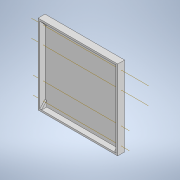
# Autodesk Inventor part: Bottom Base
Saved by Autodesk Inventor 2022 (Build 260153000, 153)
## iProperties
Created: 2022-04-03
Part Number: Bottom Base
Material: Generic
Document SubType Name: Modeling
Designer: Nick
Density: 1 g/cm^3
Appearance: Default
Author: Nick
Autodesk Inventor part; units mm, degrees
ref_plane "YZ Plane" through (0, 0, 0) normal (1, 0, 0) x (0, 1, 0)
ref_plane "XZ Plane" through (0, 0, 0) normal (0, 1, 0) x (-1, 0, 0)
ref_plane "XY Plane" through (0, 0, 0) normal (0, 0, 1) x (1, 0, 0)
sketch "Sketch1" plane through (0, 0, 0) normal (0, 0, 1) x (1, 0, 0)
  line L0 (0, 0) -> (292.1, 0)
  line L1 (292.1, 0) -> (292.1, 292.1)
  line L2 (292.1, 292.1) -> (0, 292.1)
  line L3 (0, 292.1) -> (0, 0)
  dimension "d11" = 292.1
  dimension "d12" = 292.1
  constraints: 8 end point, 2 parallel, 1 horizontal, 1 perpendicular
  measures "d11" distance of L2.end L1.end
  measures "d12" distance of L1.end L0.end
extrude "Extrusion3" add sketch "Sketch1" along normal blind 25.4
sketch "Sketch2" plane through (0, 0, 0) normal (-1, 0, 0) x (0, 0, 1)
  line L0 (25.4, 0) -> (25.4, 292.1) projected
  line L1 (25.4, 0) -> (25.4, 88.9)
  line L2 (25.4, 292.1) -> (25.4, 203.2)
  point P0 (0, 0)
  dimension "d15" = 88.9
  dimension "d16" = 88.9
  constraints: 4 end point, 2 coincident, 2 point on line
  measures "d15" distance of L0.start L1.end
  measures "d16" distance of L0.end L2.end
shell "Shell1" thickness 6.35 removed faces 1 at (97.3667, 194.7333, 25.4)
sketch "Sketch3" plane through (6.35, 6.35, 6.35) normal (1, 0, 0) x (0, 0, -1)
  line L0 (0, 279.4) -> (0, 0) projected
  line L1 (0, 279.4) -> (-19.05, 279.4) projected
  line L2 (-19.05, 0) -> (-19.05, 279.4) projected
  line L3 (0, 0) -> (-19.05, 0) projected
  line L4 (0, 279.4) -> (-19.05, 279.4) projected
  line L5 (-19.05, 260.35) -> (0, 260.35) construction
  line L6 (0, 279.4) -> (0, 0) projected
  line L7 (6.35, 285.75) -> (-19.05, 285.75) projected
  line L8 (6.35, -6.35) -> (-19.05, -6.35) projected
  point P0 (-6.35, 260.35)
  point P1 (-6.35, 196.85)
  point P2 (-6.35, 82.55)
  point P3 (-6.35, 19.05)
  dimension "d20" = 25.4
  dimension "d21" = 12.7
  dimension "d22" = 88.9
  dimension "d23" = 88.9
  dimension "d24" = 25.4
  constraints: 3 point on line, 3 vertical alignment, 2 end point, 1 perpendicular
  measures "d20" distance between parallel lines of L5 L7
  measures "d21" distance from line of L2 point (-6.35, 260.35)
  measures "d22" distance from line of L7 point (-6.35, 196.85)
  measures "d23" distance from line of L8 point (-6.35, 82.55)
  measures "d24" distance from line of L8 point (-6.35, 19.05)
sketch "Sketch4" plane through (285.75, 6.35, 6.35) normal (-1, 0, 0) x (0, 0, 1)
  line L0 (0, 0) -> (0, 279.4) projected
  line L1 (0, 0) -> (19.05, 0) projected
  line L2 (19.05, 279.4) -> (19.05, 0) projected
  line L3 (0, 279.4) -> (19.05, 279.4) projected
  line L4 (19.05, 0) -> (0, 21.4113)
  line L5 (0, 0) -> (0, 279.4) projected
  point P0 (-6.35, -6.35)
  point P1 (0, 21.4113)
  dimension "d25" = 41.66
  constraints: 2 end point, 1 point on line
  measures "d25" angle of L4 L0
extrude "Extrusion4" add sketch "Sketch4" along normal blind 6.35 contours L0 L4 L1
ref_plane "Work Plane1" through (146.05, 0, 0) normal (-1, 0, 0) x (0, 0, 1)
ref_plane "Work Plane2" through (0, 146.05, 0) normal (0, 1, 0) x (1, 0, 0)
mirror "Mirror1" about plane through (146.05, 0, 0) normal (-1, 0, 0) of "Extrusion4"
mirror "Mirror2" about plane through (0, 146.05, 0) normal (0, 1, 0) of "Extrusion4", "Mirror1"
equation "\"d23\" = d22"
equation "\"d24\" = d20"
body "Solid2"
